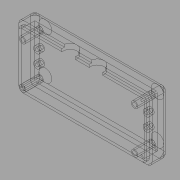
# Autodesk Inventor part: case_bottom
Saved by Autodesk Inventor 2013 (Build 170138000, 138)
## iProperties
Created: 2014-06-07
Part Number: case_bottom
Material: Generic
Document SubType Name: Modeling
Designer: Brad
Density: 1 g/cm^3
Author: Brad
Autodesk Inventor part; units mm, degrees
ref_plane "YZ Plane" through (0, 0, 0) normal (1, 0, 0) x (0, 1, 0)
ref_plane "XZ Plane" through (0, 0, 0) normal (0, 1, 0) x (-1, 0, 0)
ref_plane "XY Plane" through (0, 0, 0) normal (0, 0, 1) x (1, 0, 0)
sketch "Sketch1" plane through (0, 0, 0) normal (0, 0, 1) x (1, 0, 0)
  line L0 (-48.26, 22.86) -> (48.26, 22.86)
  line L1 (48.26, 22.86) -> (48.26, -22.86)
  line L2 (48.26, -22.86) -> (-48.26, -22.86)
  line L3 (-48.26, -22.86) -> (-48.26, 22.86)
  line L4 (-44.45, 19.05) -> (44.45, 19.05)
  line L5 (44.45, 19.05) -> (44.45, -19.05)
  line L6 (44.45, -19.05) -> (-44.45, -19.05)
  line L7 (-44.45, -19.05) -> (-44.45, 19.05)
  point P0 (0, 0)
  dimension "d0" = 88.9
  dimension "d3" = 38.1
  dimension "d4" = 19.05
  dimension "d5" = 44.45
  dimension "d8" = 3.81
  dimension "d9" = 3.81
  dimension "d10" = 3.81
  dimension "d11" = 3.81
  constraints: 16 end point, 4 parallel, 2 horizontal, 2 perpendicular
  measures "d0" distance of L4.start L4.end
  measures "d3" distance of L4.end L5.end
  measures "d4" distance from line of point (0, 0) L4
  measures "d5" distance from line of point (0, 0) L5
  measures "d8" distance between parallel lines of L5 L1
  measures "d9" distance between parallel lines of L0 L4
  measures "d10" distance between parallel lines of L7 L3
  measures "d11" distance between parallel lines of L2 L6
extrude "Extrusion1" add sketch "Sketch1" along normal blind 7.7343
sketch "Sketch2" plane through (0, 0, 0) normal (0, 0, -1) x (-1, 0, 0)
  line L0 (48.26, 22.86) -> (-48.26, 22.86) projected
  line L1 (-48.26, -22.86) -> (48.26, -22.86) projected
  line L2 (48.26, -22.86) -> (48.26, 22.86) projected
  line L3 (-48.26, 22.86) -> (48.26, 22.86)
  line L4 (48.26, 22.86) -> (48.26, -22.86)
  line L5 (48.26, -22.86) -> (-48.26, -22.86)
  line L6 (-48.26, 22.86) -> (-48.26, -22.86)
  point P0 (0, 0)
  constraints: 8 end point, 3 perpendicular, 1 collinear
extrude "Extrusion2" add sketch "Sketch2" along normal blind 3.81
sketch "Sketch3" plane through (0, 0, 0) normal (0, 0, 1) x (1, 0, 0)
  circle A0 centre (-39.6875, -4.7625) radius 2.413
  circle A1 centre (39.6875, -4.7625) radius 2.413
  circle A2 centre (-39.6875, 4.7625) radius 2.413
  circle A3 centre (39.6875, 4.7625) radius 2.413
  point P0 (0, 0)
  dimension "d16" = 79.375
  dimension "d18" = 39.6875
  dimension "d19" = 4.826
  dimension "d20" = 4.826
  dimension "d21" = 79.375
  dimension "d22" = 4.826
  dimension "d23" = 4.826
  dimension "d24" = 9.525
  dimension "d25" = 4.7625
  constraints: 4 centre point
  measures "d16" distance of A1.centre A0.centre
  measures "d18" horizontal distance of point (0, 0) A0.centre
  measures "d19" diameter of A0
  measures "d20" diameter of A1
  measures "d21" distance of A3.centre A2.centre
  measures "d22" diameter of A2
  measures "d23" diameter of A3
  measures "d24" distance of A0.centre A2.centre
  measures "d25" vertical distance of point (0, 0) A0.centre
extrude "Extrusion3" add sketch "Sketch3" along normal blind 3.302
sketch "Sketch4" plane through (-39.6875, -4.7625, 3.302) normal (0, 0, 1) x (1, 0, 0)
  circle A0 centre (0, 0) radius 2.413 projected
  circle A1 centre (0, 0) radius 1.143
  point P0 (39.6875, 4.7625)
  dimension "d28" = 2.286
  constraints: 1 centre point, 1 coincident
  measures "d28" diameter of A1
sketch "Sketch5" plane through (-39.6875, 4.7625, 3.302) normal (0, 0, 1) x (1, 0, 0)
  circle A0 centre (0, 0) radius 1.143
  point P0 (39.6875, 4.7625)
  dimension "d30" = 2.286
  constraints: 1 centre point
  measures "d30" diameter of A0
sketch "Sketch6" plane through (39.6875, 4.7625, 3.302) normal (0, 0, 1) x (1, 0, 0)
  circle A0 centre (0, 0) radius 1.143
  point P0 (39.6875, 4.7625)
  dimension "d31" = 2.286
  constraints: 1 centre point
  measures "d31" diameter of A0
sketch "Sketch7" plane through (39.6875, -4.7625, 3.302) normal (0, 0, 1) x (1, 0, 0)
  circle A0 centre (0, 0) radius 1.143
  point P0 (39.6875, 4.7625)
  dimension "d32" = 2.286
  constraints: 1 centre point
  measures "d32" diameter of A0
extrude "Extrusion4" cut sketch "Sketch4" against normal blind 3.556 contours A1
extrude "Extrusion5" cut sketch "Sketch5" against normal blind 3.556
extrude "Extrusion6" cut sketch "Sketch6" against normal blind 3.556
extrude "Extrusion7" cut sketch "Sketch7" against normal blind 3.556
sketch "Sketch8" plane through (0, 0, 0) normal (0, 0, 1) x (1, 0, 0)
  line L0 (44.45, 19.05) -> (-44.45, 19.05) projected
  line L1 (-44.45, 19.05) -> (-44.45, -19.05) projected
  line L2 (-44.45, -19.05) -> (44.45, -19.05) projected
  circle A0 centre (-40.64, 15.24) radius 2.3495
  line L3 (0, 0) -> (0, 6.0691)
  line L4 (0, 0) -> (-4.9329, 0)
  circle A1 centre (40.64, 15.24) radius 2.3495
  circle A2 centre (-40.64, -15.24) radius 2.3495
  circle A3 centre (40.64, -15.24) radius 2.3495
  dimension "d41" = 4.699
  dimension "d42" = 3.81
  dimension "d43" = 3.81
  constraints: 4 centre point, 4 end point, 3 symmetric about line, 2 perpendicular, 3 other
  measures "d41" diameter of A0
  measures "d42" distance from line of L1 A0.centre
  measures "d43" distance from line of L0 A0.centre
extrude "Extrusion8" add sketch "Sketch8" along normal blind 12.7
sketch "Sketch9" plane through (0, 0, 7.7343) normal (0, 0, 1) x (1, 0, 0)
  line L0 (44.45, 19.05) -> (44.45, -19.05) projected
  line L1 (44.45, -19.05) -> (-44.45, -19.05) projected
  line L2 (-44.45, -19.05) -> (-44.45, 19.05) projected
  line L3 (-44.45, 19.05) -> (44.45, 19.05) projected
  line L4 (48.26, 22.86) -> (-48.26, 22.86) projected
  line L5 (-46.355, 20.955) -> (46.355, 20.955)
  line L6 (46.355, 20.955) -> (46.355, -20.955)
  line L7 (46.355, -20.955) -> (-46.355, -20.955)
  line L8 (-46.355, -20.955) -> (-46.355, 20.955)
  line L9 (44.45, -19.05) -> (-44.45, -19.05)
  line L10 (-44.45, -19.05) -> (-44.45, 19.05)
  line L11 (-44.45, 19.05) -> (44.45, 19.05)
  line L12 (44.45, 19.05) -> (44.45, -19.05)
  point P0 (0, 0)
  dimension "d46" = 1.905
  dimension "d48" = 3.81
  dimension "d49" = 1.905
  dimension "d50" = 1.905
  dimension "d51" = 1.905
  constraints: 16 end point, 4 parallel, 2 horizontal, 2 perpendicular
  measures "d46" distance between parallel lines of L5 L11
  measures "d48" distance between parallel lines of L4 L3
  measures "d49" distance between parallel lines of L8 L2
  measures "d50" distance between parallel lines of L6 L0
  measures "d51" distance between parallel lines of L7 L1
extrude "Extrusion9" add sketch "Sketch9" along normal blind 1.905
sketch "Sketch10" plane through (0, 0, 0) normal (0, 0, 1) x (1, 0, 0)
  circle A0 centre (-40.64, 15.24) radius 2.3495 projected
  line L0 (44.45, 19.05) -> (-44.45, 19.05) projected
  line L1 (-44.45, 19.05) -> (-44.45, -19.05) projected
  arc A1 (-41.9028, 17.2213) -> (-42.6213, 16.5028) centre (-40.64, 15.24) ccw
  line L2 (-44.45, 19.05) -> (-43.7316, 19.05)
  line L3 (-44.45, 19.05) -> (-44.45, 19.05)
  line L4 (-44.45, 18.3316) -> (-42.6213, 16.5028)
  line L5 (-43.7316, 19.05) -> (-41.9028, 17.2213)
  line L6 (-44.45, 19.05) -> (-42.6578, 17.2578)
  line L7 (-44.45, 19.05) -> (-43.7316, 19.05)
  line L8 (-44.45, 18.3316) -> (-44.45, 19.05)
  line L9 (0, 0) -> (0, 5.3825)
  line L10 (0, 0) -> (-5.6374, 0)
  arc A2 (42.6213, 16.5028) -> (41.9028, 17.2213) centre (40.64, 15.24) ccw
  line L11 (44.45, 18.3316) -> (42.6213, 16.5028)
  line L12 (43.7316, 19.05) -> (41.9028, 17.2213)
  line L13 (44.45, 19.05) -> (43.7316, 19.05)
  line L14 (44.45, 18.3316) -> (44.45, 19.05)
  line L15 (44.45, -18.3316) -> (42.6213, -16.5028)
  line L16 (44.45, -18.3316) -> (44.45, -19.05)
  line L17 (44.45, -19.05) -> (43.7316, -19.05)
  line L18 (43.7316, -19.05) -> (41.9028, -17.2213)
  arc A3 (41.9028, -17.2213) -> (42.6213, -16.5028) centre (40.64, -15.24) ccw
  arc A4 (-42.6213, -16.5028) -> (-41.9028, -17.2213) centre (-40.64, -15.24) ccw
  line L19 (-43.7316, -19.05) -> (-41.9028, -17.2213)
  line L20 (-44.45, -18.3316) -> (-42.6213, -16.5028)
  line L21 (-44.45, -18.3316) -> (-44.45, -19.05)
  line L22 (-44.45, -19.05) -> (-43.7316, -19.05)
  point P0 (44.45, -19.05)
  point P1 (-44.45, -19.05)
  dimension "d54" = 45
  dimension "d55" = 45
  dimension "d56" = 1.016
  dimension "d57" = 0.508
  dimension "d58" = 0.508
  constraints: 42 end point, 21 symmetric about line, 10 point on circle, 4 centre point, 2 parallel, 2 point on line, 1 coincident, 1 collinear, 1 concentric, 1 perpendicular, 3 other
  measures "d54" angle of L4 L3
  measures "d55" angle of L0 L5
  measures "d56" distance between parallel lines of L5 L4
  measures "d57" distance between parallel lines of L5 L6
  measures "d58" distance between parallel lines of L4 L6
extrude "Extrusion10" add sketch "Sketch10" along normal blind 9.6393 contours L14 L11 A2 L12 L0 | L20 A4 L19 L22 L1 | L16 L17 L18 A3 L15
sketch "Sketch11" plane through (0, 0, -3.81) normal (0, 0, -1) x (-1, 0, 0)
  line L0 (48.26, -22.86) -> (48.26, 22.86) projected
  circle A0 centre (-40.64, 15.24) radius 1.4605
  arc A1 (-42.6213, 16.5028) -> (-41.9028, 17.2213) centre (-40.64, 15.24) ccw projected
  line L1 (-7.4922, 0) -> (0, 0)
  line L2 (0, 0) -> (0, 6.6008)
  circle A2 centre (40.64, 15.24) radius 1.4605
  circle A3 centre (-40.64, -15.24) radius 1.4605
  circle A4 centre (40.64, -15.24) radius 1.4605
  dimension "d61" = 2.921
  constraints: 4 centre point, 4 end point, 3 symmetric about line, 2 perpendicular, 1 concentric, 3 other
  measures "d61" diameter of A0
extrude "Extrusion11" cut sketch "Sketch11" against normal blind 16.51
chamfer "Chamfer1" distance 3.175 angle 45 4 edges at (42.1005, 15.24, -3.81) (42.1005, -15.24, -3.81) (-39.1795, -15.24, -3.81) (-39.1795, 15.24, -3.81)
fillet "Fillet1" radius 3.175 8 edges at (46.355, 20.955, 8.6868) (48.26, 22.86, 1.9621) (48.26, -22.86, 1.9621) (-46.355, 20.955, 8.6868) (-48.26, 22.86, 1.9621) (-48.26, -22.86, 1.9621) (-46.355, -20.955, 8.6868) (46.355, -20.955, 8.6868)
fillet "Fillet2" radius 3.175 8 edges at (47.3301, 21.9301, -3.81) (48.26, 0, -3.81) (47.3301, -21.9301, -3.81) (0, -22.86, -3.81) (-47.3301, -21.9301, -3.81) (-48.26, 0, -3.81) (-47.3301, 21.9301, -3.81) (0, 22.86, -3.81)
sketch "Sketch12" plane through (-44.45, 19.05, 0) normal (0, -1, 0) x (1, 0, 0)
  line L0 (88.1816, 0) -> (88.1816, 9.6393) projected
  line L1 (88.1816, 0) -> (0, 0) projected
  line L2 (0, 9.6393) -> (88.1816, 9.6393)
  line L3 (44.0872, 9.6393) -> (44.0872, 5.2149)
  circle A0 centre (34.2447, 8.6868) radius 5
  line L4 (-0.0072, 0) -> (88.1744, 0)
  circle A1 centre (53.9297, 8.6868) radius 5
  line L5 (0, 0) -> (0, 9.6393) projected
  point P0 (44.45, 0)
  dimension "d70" = 88.1816
  dimension "d71" = 44.0944
  dimension "d72" = 9.8425
  dimension "d73" = 8.6868
  dimension "d74" = 10
  dimension "d77" = 9.8425
  dimension "d78" = 44.0872
  constraints: 6 end point, 3 symmetric about line, 2 centre point, 2 perpendicular, 1 point on line, 1 other
  measures "d70" distance of L2.start L0.end
  measures "d71" distance between parallel lines of L0 L3
  measures "d72" distance from line of L3 A0.centre
  measures "d73" distance from line of L1 A0.centre
  measures "d74" diameter of A0
  measures "d77" distance from line of L3 A1.centre
  measures "d78" distance between parallel lines of L5 L3
extrude "Extrusion12" cut sketch "Sketch12" against normal blind 5.08 contours A1 L2 | L2 A1 | A0 L2 | L2 A0
body "Solid1"
